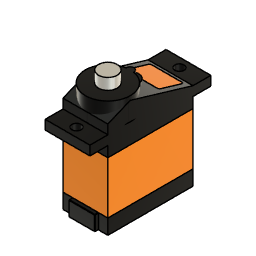
Savöx_SH_0255 MG_micro_servo (Autodesk Fusion 360 design; units mm, degrees)
Autodesk Fusion 360 part; units mm, degrees
note: some values were not read from the file. Chosen so that the rebuilt part matches the saved one: which bodies a step acts on; a direction. Set by a fixed rule: which sketch regions a step uses.
sketch "Side Profile" plane through (0, 0, 0) normal (1, 0, 0) x (0, 1, 0)
  line L0 (0, 0) -> (22.8, 0)
  line L1 (22.8, 0) -> (22.8, 20.82)
  line L2 (22.8, 20.82) -> (27.6, 20.82)
  line L3 (0, 25.82) -> (0, 23.32)
  line L4 (0, 23.32) -> (-4.8, 23.32)
  line L5 (-4.8, 23.32) -> (-4.8, 20.82)
  line L6 (-4.8, 20.82) -> (0, 20.82)
  line L7 (0, 20.82) -> (0, 0)
  line L8 (0, 25.82) -> (6, 28.32)
  line L9 (6, 28.32) -> (22.8, 23.32)
  line L10 (27.6, 20.82) -> (27.6, 23.32)
  line L11 (27.6, 23.32) -> (22.8, 23.32)
  dimension "d1" = 22.8
  dimension "d3" = 20.82
  dimension "d4" = 20.82
  dimension "d6" = 2.5
  dimension "d10" = 4.8
  dimension "d25" = 2.5
  dimension "d26" = 6
  dimension "d27" = 2.5
  dimension "d28" = 2.5
  dimension "d29" = 4.8
  dimension "d48" = 32.4
  constraint coincident L0.start L7.end
  constraint horizontal L0
  constraint perpendicular L0 L1
  constraint perpendicular L1 L2
  constraint perpendicular L4 L5
  constraint perpendicular L5 L6
  constraint perpendicular L0 L7
  constraint collinear L3 L7
  constraint perpendicular L2 L10
  constraint perpendicular L10 L11
  measures "d1" distance of L0.start L0.end
  measures "d3" distance of L0.end L1.end
  measures "d4" distance of L6.end L0.start
  measures "d6" distance of L4.end L5.end
  measures "d10" distance of L3.end L4.end
  measures "d25" distance of L3.start L3.end
  measures "d26" horizontal distance of L3.start L8.end
  measures "d27" vertical distance of L3.start L8.end
  measures "d28" distance of L2.end L10.end
  measures "d29" distance of L9.end L10.end
  measures "d48" distance of L5 L10
extrude "Extrude1" add sketch "Side Profile" along normal blind 12 makes body 1
sketch "Aluminium and Plastic Segments" plane through (12, 0, 0) normal (1, 0, 0) x (0, 1, 0)
  line L0 (0, 25.82) -> (0, 23.32)
  line L1 (0, 23.32) -> (-4.8, 23.32)
  line L2 (-4.8, 23.32) -> (-4.8, 20.82)
  line L3 (-4.8, 20.82) -> (0, 20.82)
  line L4 (0, 20.82) -> (0, 0)
  line L5 (0, 0) -> (22.8, 0)
  line L6 (22.8, 0) -> (22.8, 20.82)
  line L7 (22.8, 20.82) -> (27.6, 20.82)
  line L8 (27.6, 20.82) -> (27.6, 23.32)
  line L9 (27.6, 23.32) -> (22.8, 23.32)
  line L10 (22.8, 23.32) -> (6, 28.32)
  line L11 (6, 28.32) -> (0, 25.82)
  line L12 (0, 0) -> (22.8, 0)
  line L13 (22.8, 0) -> (22.8, 4)
  line L14 (22.8, 4) -> (0, 4)
  line L15 (0, 4) -> (0, 0)
  line L16 (0, 4) -> (22.8, 4)
  line L17 (22.8, 4) -> (22.8, 18)
  line L18 (22.8, 18) -> (0, 18)
  line L19 (0, 18) -> (0, 4)
  dimension "d30" = 4
  dimension "d31" = 14
  constraint horizontal L12
  constraint vertical L13
  constraint horizontal L14
  constraint vertical L15
  constraint coincident L6 L13.end
  constraint coincident L4.end L5.start
  constraint horizontal L16
  constraint vertical L17
  constraint horizontal L18
  constraint vertical L19
  measures "d30" distance of L4.end L14.end
  measures "d31" distance of L14.end L18.end
copy_body "CopyPasteBodies2" bodies 1 makes body 2
extrude "Extrude5" cut sketch "Aluminium and Plastic Segments" against normal blind 12 contours L4 L6 L14 L16 L17 L18 L19 bodies 1 makes body 3 at (4, 7.6, 18)
extrude "Extrude6" cut sketch "Aluminium and Plastic Segments" against normal blind 12 contours L0 L1 L2 L3 L4 L6 L7 L8 L9 L10 L11 L18 | L4 L5 L6 L12 L13 L14 L15 L16 bodies 2
sketch "Label" plane through (0, 8.231, 27.656) normal (0, 0.285254, 0.958452) x (-1, 0, 0)
  line L0 (0, -15.2006) -> (0, 2.3277)
  line L1 (0, 2.3277) -> (-12, 2.3277)
  line L2 (-12, 2.3277) -> (-12, -15.2006)
  line L3 (-12, -15.2006) -> (0, -15.2006)
  line L4 (-10.5, -7.2006) -> (-1.5, -7.2006)
  line L5 (-1.5, -7.2006) -> (-1.5, -14.2006)
  line L6 (-1.5, -14.2006) -> (-10.5, -14.2006)
  line L7 (-10.5, -14.2006) -> (-10.5, -7.2006)
  dimension "d38" = 9
  dimension "d39" = 7
  dimension "d40" = 1.5
  dimension "d41" = 1.5
  dimension "d43" = 1
  constraint horizontal L4
  constraint vertical L5
  constraint horizontal L6
  constraint vertical L7
  measures "d38" distance of L4.start L4.end
  measures "d39" distance of L4.start L6.end
  measures "d40" distance of L2 L7
  measures "d41" distance of L0 L5
  measures "d43" distance of L3 L6
extrude "Extrude7" add sketch "Label" along normal blind 0.01 separate body contours L4 L5 L6 L7 makes body 4
fillet "Fillet1" radius 0.5 4 edges at (10.5, 21.843, 23.61) (10.5, 15.1338, 25.6068) (1.5, 21.843, 23.61) (1.5, 15.1338, 25.6068) on bodies 4
sketch "Holes" plane through (0, 0, 23.32) normal (0, 0, 1) x (-1, 0, 0)
  line L0 (0, -27.6) -> (0, -22.8)
  line L1 (0, -22.8) -> (-12, -22.8)
  line L2 (-12, -22.8) -> (-12, -27.6)
  line L3 (-12, -27.6) -> (0, -27.6)
  line L4 (0, 0) -> (0, 4.8)
  line L5 (0, 4.8) -> (-12, 4.8)
  line L6 (-12, 4.8) -> (-12, 0)
  line L7 (-12, 0) -> (0, 0)
  circle A0 centre (-6, -25.2) radius 1.25
  circle A1 centre (-6, 2.4) radius 1.25
  dimension "d49" = 2.5
  dimension "d50" = 2.5
  dimension "d52" = 2.4
  dimension "d53" = 2.4
  dimension "d54" = 2.4
  dimension "d55" = 2.4
  dimension "d57" = 6
  dimension "d58" = 6
  dimension "d59" = 6
  dimension "d60" = 6
  dimension "d84" = 27.6
  measures "d49" diameter of A0
  measures "d50" diameter of A1
  measures "d52" distance of L1 A0.centre
  measures "d53" distance of L3 A0.centre
  measures "d54" distance of L7 A1.centre
  measures "d55" distance of L5 A1.centre
  measures "d57" distance of L0 A0.centre
  measures "d58" distance of L2 A0.centre
  measures "d59" distance of L4 A1.centre
  measures "d60" distance of L6 A1.centre
  measures "d84" distance of A0.centre A1.centre
extrude "Extrude8" cut sketch "Holes" against normal blind 2.5 contours A0 | A1 bodies 3
sketch "Top Cylinders" plane through (0, 0, 23.32) normal (0, 0, 1) x (-1, 0, 0)
  circle A0 centre (-6, -25.2) radius 1.25
  line L0 (0, -27.6) -> (0, -22.8)
  line L1 (0, -22.8) -> (-12, -22.8)
  line L2 (-12, -22.8) -> (-12, -27.6)
  line L3 (-12, -27.6) -> (0, -27.6)
  line L4 (0, -6) -> (0, 0)
  line L5 (0, 0) -> (-12, 0)
  line L6 (-12, 0) -> (-12, -6)
  line L7 (-12, -6) -> (0, -6)
  line L8 (0, -22.8) -> (0, -6)
  line L9 (0, -6) -> (-12, -6)
  line L10 (-12, -6) -> (-12, -22.8)
  line L11 (-12, -22.8) -> (0, -22.8)
  circle A1 centre (-6, -6) radius 6
  circle A2 centre (-6, -12) radius 2.25
  dimension "d63" = 12
  dimension "d68" = 4.5
  dimension "d69" = 6
  constraint tangent L5 A1
  constraint tangent L8 A1
  constraint coincident A1 A2.centre
  measures "d63" diameter of A1
  measures "d68" diameter of A2
  measures "d69" distance of L10 A2.centre
extrude "Extrude9" add sketch "Top Cylinders" along normal blind 6.08 separate body contours L7 L9 A1 A2 | L7 L9 A1 | A1 A2 | A1 A2 makes body 5
sketch "Small Top Cylinder" plane through (0, 0, 29.4) normal (0, 0, 1) x (-1, 0, 0)
  arc A0 (-8.2101, -11.5781) -> (-3.7899, -11.5781) centre (-6, -12) ccw
  arc A1 (-3.7899, -11.5781) -> (-8.2101, -11.5781) centre (-6, -6) ccw
  circle A2 centre (-6, -6) radius 6
  circle A3 centre (-6, -12) radius 1
  dimension "d70" = 12
  dimension "d71" = 2
  constraint concentric A1 A2
  constraint concentric A0 A3
  measures "d70" diameter of A2
  measures "d71" diameter of A3
extrude "Extrude10" cut sketch "Small Top Cylinder" against normal blind 2 contours A0 A2 A3 bodies 5
sketch "Cable Port" plane through (0, 0, 0) normal (0, -1, 0) x (1, 0, 0)
  line L0 (12, 4) -> (0, 4)
  line L1 (0, 4) -> (0, 0)
  line L2 (0, 0) -> (12, 0)
  line L3 (12, 0) -> (12, 4)
  line L4 (2.5, 4) -> (9.5, 4)
  line L5 (9.5, 4) -> (9.5, 0)
  line L6 (9.5, 0) -> (2.5, 0)
  line L7 (2.5, 0) -> (2.5, 4)
  dimension "d74" = 7
  dimension "d75" = 2.5
  dimension "d76" = 2.5
  constraint horizontal L4
  constraint vertical L5
  constraint horizontal L6
  constraint vertical L7
  constraint coincident L0 L4.start
  measures "d74" distance of L4.start L4.end
  measures "d75" distance of L1 L7
  measures "d76" distance of L3 L5
extrude "Extrude11" add sketch "Cable Port" along normal blind 1 contours L0 L2 L4 L5 L6 L7 bodies 1
fillet "Fillet2" radius 0.1 8 edges at (9.5, -0.5, 4) (6, -1, 4) (9.5, -1, 2) (6, -1, 0) (2.5, -1, 2) (9.5, -0.5, 0) (2.5, -0.5, 4) (2.5, -0.5, 0) on bodies 1
sketch "Turning Gear" plane through (0, 0, 29.4) normal (0, 0, 1) x (-1, 0, 0)
  arc A0 (-5.0035, -11.9167) -> (-6.9965, -11.9167) centre (-6, -6) ccw
  arc A1 (-6.9965, -11.9167) -> (-5.0035, -11.9167) centre (-6, -12) ccw
  circle A2 centre (-6, -6) radius 2.5
  dimension "d81" = 5
  constraint concentric A0 A2
  measures "d81" diameter of A2
extrude "Extrude12" add sketch "Turning Gear" along normal blind 3 separate body contours A2 makes body 6
named bodies: "Servo Motor Body Bottom", "Servo Motor Body Plastic", "Servo Motor Body Middle", "Servo Motor Body Top", "Label", "Top Cylinders", "Turning Gear"
